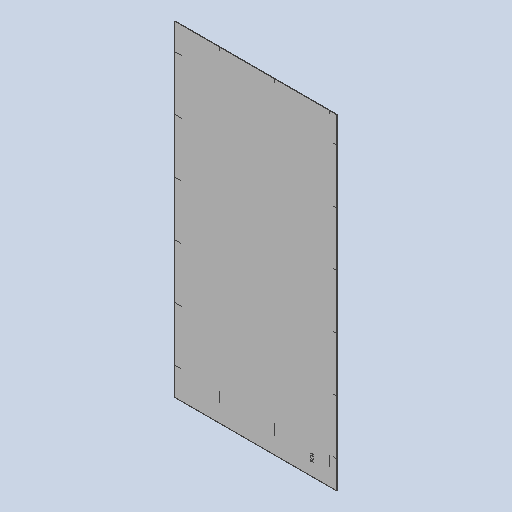
# Autodesk Inventor part: GBK 1126 shield 1.2
Saved by Autodesk Inventor 2026.2 (Build 302298000, 298)
## iProperties
Manager: 10
Created: 2026-04-17
Part Number: GBK 1126 shield 1.2
Material: Steel
Document SubType Name: Sheet Metal
Designer: admin
Stock Number: 1126
Mass: 138487 g
Surface Area: 88564.8 cm^2
Volume: 17641.6 cm^3
Density: 7.85 g/cm^3
Flat Pattern Width: 148 cm
Flat Pattern Length: 298 cm
Flat Pattern Area: 44104 cm^2
Sheet Metal Rule: Default_mm
Sheet Metal Width: 1480,000 мм
Sheet Metal Length: 2980,000 мм
Sheet Metal Area: 4410400,000 мм^2
Appearance: Default
Description: правим
Project: правим ++
Author: admin
Revision Number: 10
Comments: !!!
Autodesk Inventor part; units mm, degrees
ref_plane "YZ Plane" through (0, 0, 0) normal (1, 0, 0) x (0, 1, 0)
ref_plane "XZ Plane" through (0, 0, 0) normal (0, 1, 0) x (-1, 0, 0)
ref_plane "XY Plane" through (0, 0, 0) normal (0, 0, 1) x (1, 0, 0)
sketch "Sketch1" plane through (0, 0, 0) normal (0, 0, 1) x (1, 0, 0)
  line L0 (740, -1490) -> (-740, -1490)
  line L1 (-740, -1490) -> (-740, 1490)
  line L2 (-740, 1490) -> (740, 1490)
  line L3 (740, 1490) -> (740, -1490)
  line L4 (740, -1490) -> (-740, 1490) construction
  line L5 (-740, -1490) -> (740, 1490) construction
  point P0 (0, 0)
  dimension "d0" = 1480
  dimension "d1" = 2980
  measures "d0" distance of L1.end L2.end
  measures "d1" distance of L0.end L1.end
extrude "Plate2" add sketch "Sketch1" along normal blind 4
sketch "Sketch4" plane through (0, 0, 4) normal (0, 0, 1) x (1, 0, 0)
  line L0 (528.5199, -1299.683) -> (528.5199, -1657.3735) construction
  line L1 (528.5199, -1657.3735) -> (497.2557, -1657.3735) construction
  line L2 (497.2557, -1657.3735) -> (497.2557, -1299.683) construction
  line L3 (497.2557, -1299.683) -> (528.5199, -1299.683) construction
  line L4 (669.8628, -1238) -> (669.8628, -1335) projected
  line L5 (669.8628, -1335) -> (665.8638, -1335) projected
  line L6 (169.7342, -1238) -> (169.7342, -1335) projected
  line L7 (169.7342, -1335) -> (165.7352, -1335) projected
  line L8 (-330.3944, -1238) -> (-330.3944, -1335) projected
  line L9 (-330.3944, -1335) -> (-334.3934, -1335) projected
  ellipse E0 centre (-330.3944, 1490.5) end of major axis (-330.3944, 1520.5) minor radius 0.6803 (-330.3944, 1460.5) -> (-330.3944, 1520.5) ccw projected
  line L10 (-330.3944, 1460.5) -> (-334.3934, 1460.5) projected
  ellipse E1 centre (169.7342, 1490.5) end of major axis (169.7342, 1520.5) minor radius 0.6803 (169.7342, 1460.5) -> (169.7342, 1520.5) ccw projected
  line L11 (169.7342, 1460.5) -> (165.7352, 1460.5) projected
  ellipse E2 centre (669.8628, 1490.5) end of major axis (669.8628, 1520.5) minor radius 0.6803 (669.8628, 1460.5) -> (669.8628, 1520.5) ccw projected
  line L12 (669.8628, 1460.5) -> (665.8638, 1460.5) projected
  line L13 (710, -1234.5) -> (770, -1234.5) projected
  line L14 (710, -1234.5) -> (710, -1230.5) projected
  line L15 (710, -737.8333) -> (770, -737.8333) projected
  line L16 (710, -737.8333) -> (710, -733.8333) projected
  line L17 (710, -241.1667) -> (770, -241.1667) projected
  line L18 (710, -241.1667) -> (710, -237.1667) projected
  line L19 (710, 255.5) -> (770, 255.5) projected
  line L20 (710, 255.5) -> (710, 259.5) projected
  line L21 (710, 752.1667) -> (770, 752.1667) projected
  line L22 (710, 752.1667) -> (710, 756.1667) projected
  line L23 (710, 1248.8333) -> (770, 1248.8333) projected
  line L24 (710, 1248.8333) -> (710, 1252.8333) projected
  line L25 (-738.6395, -1234.5) -> (-680, -1234.5) projected
  line L26 (-680, -1234.5) -> (-680, -1230.5) projected
  line L27 (-738.6395, -737.8333) -> (-680, -737.8333) projected
  line L28 (-680, -737.8333) -> (-680, -733.8333) projected
  line L29 (-738.6395, -241.1667) -> (-680, -241.1667) projected
  line L30 (-680, -241.1667) -> (-680, -237.1667) projected
  line L31 (-738.6395, 255.5) -> (-680, 255.5) projected
  line L32 (-680, 255.5) -> (-680, 259.5) projected
  line L33 (-738.6395, 752.1667) -> (-680, 752.1667) projected
  line L34 (-680, 752.1667) -> (-680, 756.1667) projected
  line L35 (-738.6395, 1248.8333) -> (-680, 1248.8333) projected
  line L36 (-680, 1248.8333) -> (-680, 1252.8333) projected
  constraints: 5 other
mark "Mark2"
equation "\"d0\" = Лист_ширина"
equation "\"BendRadius\" = Thickness"
equation "\"d3\" = Thickness"
equation "\"BendReliefWidth\" = Thickness"
equation "\"BendReliefDepth\" = 0.5 * Thickness"
equation "\"CornerReliefSize\" = 4 * Thickness"
equation "\"MinimumRemnant\" = 2 * Thickness"
equation "\"TransitionRadius\" = BendRadius"
equation "\"JacobiRadiusSize\" = BendRadius"
equation "\"GapSize\" = Thickness"
equation "\"Лист_ширина\" = 1480"
equation "\"Thickness\" = 4"
body "Solid2"
